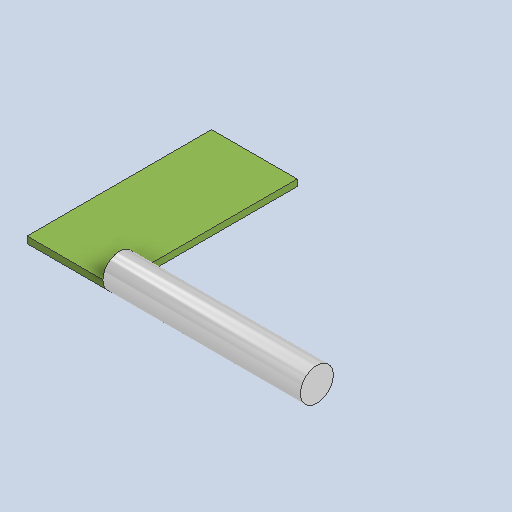
# Autodesk Inventor part: Telemetrie
Saved by Autodesk Inventor 2025.2 (Build 292293000, 293)
## iProperties
Created: 2025-03-28
Part Number: Telemetrie
Material: Generic
Document SubType Name: Modeling
Designer: mirewn
Density: 1 g/cm^3
Appearance: Default
Author: mirewn
Autodesk Inventor part; units mm, degrees
ref_plane "YZ Plane" through (0, 0, 0) normal (1, 0, 0) x (0, 1, 0)
ref_plane "XZ Plane" through (0, 0, 0) normal (0, 1, 0) x (-1, 0, 0)
ref_plane "XY Plane" through (0, 0, 0) normal (0, 0, 1) x (1, 0, 0)
sketch "Sketch1" plane through (0, 0, 0) normal (0, 1, 0) x (-1, 0, 0)
  line L0 (6.5, 14) -> (-6.5, 14)
  line L1 (-6.5, 14) -> (-6.5, -14)
  line L2 (-6.5, -14) -> (6.5, -14)
  line L3 (6.5, -14) -> (6.5, 14)
  line L4 (6.5, 14) -> (-6.5, -14) construction
  line L5 (-6.5, 14) -> (6.5, -14) construction
  point P0 (0, 0)
  dimension "d0" = 13
  dimension "d1" = 28
  constraints: 12 end point, 2 midpoint, 2 parallel, 1 horizontal, 1 perpendicular
  measures "d0" distance of L2.end L1.end
  measures "d1" distance of L1.end L0.end
extrude "Extrusion1" add sketch "Sketch1" along normal blind 1
sketch "Sketch2" plane through (6.5, 0, 14) normal (1, 0, 0) x (0, 0, -1)
  circle A0 centre (1, 1.25) radius 0.25
  circle A1 centre (1, 2.5) radius 2.5
  line L0 (0, 1) -> (28, 1) projected
  line L1 (0, 0) -> (28, 0) projected
  point P0 (14, 0)
  dimension "d4" = 0.5
  dimension "d5" = 5
  dimension "d6" = 1
  constraints: 2 centre point, 2 tangent, 1 vertical alignment
  measures "d4" diameter of A0
  measures "d5" diameter of A1
  measures "d6" horizontal distance of L0.start A0.centre
extrude "Extrusion2" add sketch "Sketch2" along normal blind 30 contours A0 | A1
body "Solid1"
